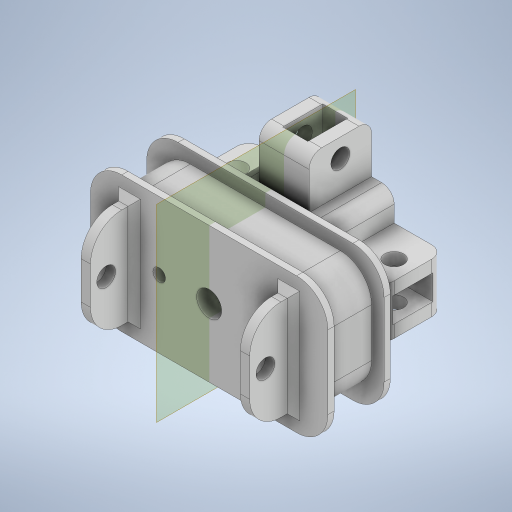
# Autodesk Inventor part: saw_end_v2
Saved by Autodesk Inventor 2024.3 (Build 283343000, 343)
## iProperties
Created: 2024-09-10
Part Number: saw_end_v2
Material: Generic
Document SubType Name: Modeling
Designer: magn1
Density: 1 g/cm^3
Appearance: Default
Author: magn1
Autodesk Inventor part; units mm, degrees
ref_plane "YZ Plane" through (0, 0, 0) normal (1, 0, 0) x (0, 1, 0)
ref_plane "XZ Plane" through (0, 0, 0) normal (0, 1, 0) x (-1, 0, 0)
ref_plane "XY Plane" through (0, 0, 0) normal (0, 0, 1) x (1, 0, 0)
sketch "Sketch1" plane through (0, 0, 0) normal (0, 0, 1) x (1, 0, 0)
  line L0 (-17, -8.875) -> (17, -8.875)
  line L1 (17, -8.875) -> (17, 8.875)
  line L2 (17, 8.875) -> (-17, 8.875)
  line L3 (-17, 8.875) -> (-17, -8.875)
  line L4 (-17, -8.875) -> (17, 8.875) construction
  line L5 (17, -8.875) -> (-17, 8.875) construction
  point P0 (0, 0)
  dimension "d0" = 34
  dimension "d1" = 17.75
  constraints: 12 end point, 2 midpoint, 2 parallel, 1 horizontal, 1 perpendicular
  measures "d0" distance of L2.end L1.end
  measures "d1" distance of L1.end L0.end
extrude "Extrusion1" add sketch "Sketch1" along normal blind 8
sketch "Sketch2" plane through (0, 0, 8) normal (0, 0, 1) x (1, 0, 0)
  line L0 (-19, -10.875) -> (19, -10.875)
  line L1 (19, -10.875) -> (19, 10.875)
  line L2 (19, 10.875) -> (-19, 10.875)
  line L3 (-19, 10.875) -> (-19, -10.875)
  line L4 (-19, -10.875) -> (19, 10.875) construction
  line L5 (19, -10.875) -> (-19, 10.875) construction
  point P0 (0, 0)
  dimension "d6" = 38
  dimension "d7" = 21.75
  constraints: 12 end point, 2 midpoint, 2 parallel, 1 horizontal, 1 perpendicular
  measures "d6" distance of L2.end L1.end
  measures "d7" distance of L1.end L0.end
extrude "Extrusion2" add sketch "Sketch2" along normal blind 1
sketch "Sketch3" plane through (0, 0, 0) normal (0, 0, -1) x (-1, 0, 0)
  line L0 (-19, 10.875) -> (19, 10.875) projected
  line L1 (-19, -10.875) -> (19, -10.875)
  line L2 (19, -10.875) -> (19, 10.875)
  line L3 (19, 10.875) -> (-19, 10.875)
  line L4 (-19, 10.875) -> (-19, -10.875)
  line L5 (-19, -10.875) -> (19, 10.875) construction
  line L6 (19, -10.875) -> (-19, 10.875) construction
  point P0 (0, 0)
  constraints: 12 end point, 2 midpoint, 2 parallel, 1 horizontal, 1 perpendicular
extrude "Extrusion3" add sketch "Sketch3" along normal blind 1
fillet "Fillet1" radius 5 12 edges at (19, 10.875, 8.5) (19, 10.875, -0.5) (19, -10.875, -0.5) (19, -10.875, 8.5) (17, -8.875, 4) (17, 8.875, 4) (-19, 10.875, 8.5) (-19, 10.875, -0.5) (-19, -10.875, -0.5) (-19, -10.875, 8.5) (-17, 8.875, 4) (-17, -8.875, 4)
sketch "Sketch6" plane through (0, 0, -1) normal (0, 0, -1) x (-1, 0, 0)
  line L0 (7.625, 8.625) -> (-7.625, 8.625)
  line L1 (-7.625, 8.625) -> (-7.625, -8.625)
  line L2 (-7.625, -8.625) -> (7.625, -8.625)
  line L3 (7.625, -8.625) -> (7.625, 8.625)
  line L4 (7.625, 8.625) -> (-7.625, -8.625) construction
  line L5 (-7.625, 8.625) -> (7.625, -8.625) construction
  circle A0 centre (0, 0) radius 2 projected
  circle A1 centre (0, 0) radius 1.5
  dimension "d19" = 15.25
  dimension "d20" = 17.25
  dimension "d21" = 3
  constraints: 12 end point, 2 midpoint, 2 parallel, 1 centre point, 1 coincident, 1 horizontal, 1 perpendicular
  measures "d19" distance of L2.end L1.end
  measures "d20" distance of L1.end L0.end
  measures "d21" diameter of A1
extrude "Extrusion6" add sketch "Sketch6" along normal blind 12 contours L3 L2 L1 L0 | A0 | A1
fillet "Fillet3" radius 2 4 edges at (-7.625, -8.625, -7) (7.625, -8.625, -7) (7.625, 8.625, -7) (-7.625, 8.625, -7)
sketch "Sketch9" plane through (0, 0, 9) normal (0, 0, 1) x (1, 0, 0)
  line L0 (0, 0) -> (12, 0) construction
  line L1 (0, 0) -> (-12, 0) construction
  line L2 (-12, 0) -> (-13.5, 0)
  line L3 (-13.5, 0) -> (-13.5, 8)
  line L4 (-13.5, 8) -> (-12, 8)
  line L5 (-12, 8) -> (-12, 0)
  line L6 (-13.5, 0) -> (-12, 0)
  line L7 (-12, 0) -> (-12, -8)
  line L8 (-12, -8) -> (-13.5, -8)
  line L9 (-13.5, -8) -> (-13.5, 0)
  line L10 (12, 0) -> (13.5, 0)
  line L11 (13.5, 0) -> (13.5, 8)
  line L12 (13.5, 8) -> (12, 8)
  line L13 (12, 8) -> (12, 0)
  line L14 (12, 0) -> (13.5, 0)
  line L15 (13.5, 0) -> (13.5, -8)
  line L16 (13.5, -8) -> (12, -8)
  line L17 (12, -8) -> (12, 0)
  dimension "d40" = 12
  dimension "d41" = 12
  dimension "d42" = 1.5
  dimension "d43" = 8
  dimension "d44" = 1.5
  dimension "d45" = 8
  dimension "d46" = 1.5
  dimension "d47" = 8
  dimension "d48" = 1.5
  dimension "d49" = 8
  constraints: 36 end point, 8 parallel, 6 horizontal, 4 perpendicular
  measures "d40" distance of L0.start L0.end
  measures "d41" distance of L0.start L1.end
  measures "d42" distance of L3.end L4.end
  measures "d43" distance of L2.end L3.end
  measures "d44" distance of L7.end L8.end
  measures "d45" distance of L6.end L7.end
  measures "d46" distance of L12.end L11.end
  measures "d47" distance of L11.end L10.end
  measures "d48" distance of L15.end L16.end
  measures "d49" distance of L14.end L15.end
extrude "Extrusion9" add sketch "Sketch9" along normal blind 7
sketch "Sketch11" plane through (13.5, -8, 9) normal (1, 0, 0) x (0, 0, -1)
  line L0 (-7, 16) -> (-7, 0) projected
  line L1 (-7, 8) -> (-4.5, 8) construction
  circle A0 centre (-4.5, 8) radius 1.5
  point P0 (9, 8)
  dimension "d52" = 2.5
  dimension "d53" = 3
  constraints: 2 end point, 1 centre point, 1 coincident, 1 horizontal, 1 midpoint
  measures "d52" distance of L1.start L1.end
  measures "d53" diameter of A0
extrude "Extrusion10" cut sketch "Sketch11" against normal up to surface (27 mm away)
fillet "Fillet4" radius 5 4 edges at (-12.75, 8, 16) (-12.75, -8, 16) (12.75, 8, 16) (12.75, -8, 16)
chamfer "Chamfer1" distance 1 angle 45 8 edges at (-13.5, 0, 9) (-12.75, -8, 9) (-12, 0, 9) (-12.75, 8, 9) (13.5, 0, 9) (12.75, 8, 9) (12, 0, 9) (12.75, -8, 9)
sketch "Sketch12" plane through (0, 0, 9) normal (0, 0, 1) x (1, 0, 0)
  circle A0 centre (0, 0) radius 2
  line L0 (0, 0) -> (8, 0) construction
  line L1 (0, 0) -> (-8, 0) construction
  circle A1 centre (-8, 0) radius 1
  circle A2 centre (8, 0) radius 1
  dimension "d73" = 4
  dimension "d74" = 8
  dimension "d75" = 8
  dimension "d76" = 2
  dimension "d77" = 2
  constraints: 4 end point, 3 centre point, 3 coincident, 2 horizontal
  measures "d73" diameter of A0
  measures "d74" distance of L0.start L0.end
  measures "d75" distance of L0.start L1.end
  measures "d76" diameter of A1
  measures "d77" diameter of A2
extrude "Extrusion11" cut sketch "Sketch12" against normal blind 6 contours A0
sketch "Sketch13" plane through (0, 0, -13) normal (0, 0, -1) x (-1, 0, 0)
  circle A0 centre (0, 0) radius 1.5
  dimension "d80" = 3
  constraints: 1 centre point, 1 coincident
  measures "d80" diameter of A0
extrude "Extrusion12" cut sketch "Sketch13" against normal blind 6
sketch "Sketch14" plane through (0, 0, -7) normal (0, 0, -1) x (-1, 0, 0)
  circle A0 centre (0, 0) radius 1.5
  dimension "d87" = 3
  constraints: 1 centre point, 1 coincident
  measures "d87" diameter of A0
loft "Loft2" cut profiles "Sketch14", "Sketch12" contours all / A2
loft "Loft3" cut profiles "Sketch14", "Sketch12" contours all / A1
sketch "Sketch15" plane through (-5.625, 8.625, -1) normal (0, 1, 0) x (1, 0, 0)
  line L0 (4.125, 12) -> (7.125, 12) construction
  line L1 (5.625, 12) -> (5.625, 2) construction
  line L2 (5.625, 6) -> (5.625, 3.1765) construction
  line L3 (5.625, 7) -> (2.625, 7) construction
  line L4 (5.625, 7) -> (8.625, 7) construction
  line L5 (5.625, 7) -> (8.625, 7) construction
  line L6 (1.625, 12) -> (3.625, 12)
  line L7 (3.625, 12) -> (3.625, 2)
  line L8 (3.625, 2) -> (1.625, 2)
  line L9 (1.625, 2) -> (1.625, 12)
  line L10 (1.625, 12) -> (3.625, 2) construction
  line L11 (3.625, 12) -> (1.625, 2) construction
  line L12 (9.625, 12) -> (7.625, 12)
  line L13 (7.625, 12) -> (7.625, 2)
  line L14 (7.625, 2) -> (9.625, 2)
  line L15 (9.625, 2) -> (9.625, 12)
  line L16 (9.625, 12) -> (7.625, 2) construction
  line L17 (7.625, 12) -> (9.625, 2) construction
  line L18 (1.625, 12) -> (9.625, 12)
  line L19 (9.625, 12) -> (9.625, 10.2)
  line L20 (9.625, 10.2) -> (1.625, 10.2)
  line L21 (1.625, 10.2) -> (1.625, 12)
  line L22 (1.625, 2) -> (9.625, 2)
  line L23 (9.625, 2) -> (9.625, 3.8)
  line L24 (9.625, 3.8) -> (1.625, 3.8)
  line L25 (1.625, 3.8) -> (1.625, 2)
  point P0 (5.625, -1)
  point P1 (3.625, 10.2)
  point P2 (7.625, 10.2)
  point P3 (7.625, 3.8)
  point P4 (3.625, 3.8)
  point P5 (3.625, 2)
  point P6 (7.625, 2)
  dimension "d121" = 8
  dimension "d96" = 10
  dimension "d97" = 3
  dimension "d98" = 180
  dimension "d99" = 3
  dimension "d100" = 2
  dimension "d101" = 10
  dimension "d102" = 2
  dimension "d103" = 10
  dimension "d111" = 8
  dimension "d112" = 1.8
  dimension "d113" = 8
  dimension "d114" = 1.8
  constraints: 48 end point, 8 parallel, 6 horizontal, 6 midpoint, 4 perpendicular, 3 collinear
  measures "d96" distance of L1.start L1.end
  measures "d97" distance of L3.start L3.end
  measures "d98" angle of L3 L4
  measures "d99" distance of L3.start L4.end
  measures "d100" distance of L7.end L8.end
  measures "d101" distance of L6.end L7.end
  measures "d102" distance of L14.end L13.end
  measures "d103" distance of L13.end L12.end
  measures "d111" distance of L19.end L20.end
  measures "d112" distance of L18.end L19.end
  measures "d113" distance of L24.end L23.end
  measures "d114" distance of L23.end L22.end
extrude "Extrusion13" add sketch "Sketch15" along normal blind 8 contours L6 L7 L20 L9 | L18 L13 L20 L7 | L20 L7 L24 L9 | L12 L15 L20 L13 | L24 L7 L8 L9 | L24 L13 L22 L7 | L20 L15 L24 L13 | L24 L15 L14 L13
sketch "Sketch16" plane through (4, 8.625, -3) normal (1, 0, 0) x (0, 0, -1)
  line L0 (10, 8) -> (0, 8) construction
  line L1 (5, 8) -> (5, 5) construction
  circle A0 centre (5, 5) radius 1.5
  point P0 (-3, -8.625)
  dimension "d106" = 3
  dimension "d107" = 3
  constraints: 2 end point, 1 centre point, 1 coincident, 1 midpoint, 1 vertical
  measures "d106" distance of L1.start L1.end
  measures "d107" diameter of A0
extrude "Extrusion14" cut sketch "Sketch16" against normal through all
fillet "Fillet5" radius 2 2 edges at (0, 16.625, -13) (0, 16.625, -3)
sketch "Sketch17" plane through (-7.625, -6.625, -1) normal (-1, 0, 0) x (0, 0, 1)
  line L0 (-12, 0) -> (-12, 13.25) projected
  line L1 (-12, 10.625) -> (-2, 10.625)
  line L2 (-2, 10.625) -> (-2, 8.625)
  line L3 (-2, 8.625) -> (-12, 8.625)
  line L4 (-12, 8.625) -> (-12, 10.625)
  line L5 (-12, 4.625) -> (-2, 4.625)
  line L6 (-2, 4.625) -> (-2, 2.625)
  line L7 (-2, 2.625) -> (-12, 2.625)
  line L8 (-12, 2.625) -> (-12, 4.625)
  line L9 (-12, 2.625) -> (-10.2, 2.625)
  line L10 (-10.2, 2.625) -> (-10.2, 10.625)
  line L11 (-10.2, 10.625) -> (-12, 10.625)
  line L12 (-12, 10.625) -> (-12, 2.625)
  line L13 (-2, 10.625) -> (-3.8, 10.625)
  line L14 (-3.8, 10.625) -> (-3.8, 2.625)
  line L15 (-3.8, 2.625) -> (-2, 2.625)
  line L16 (-2, 2.625) -> (-2, 10.625)
  point P0 (1, 6.625)
  point P1 (-12, 6.625)
  point P2 (-12, 2.625)
  point P3 (-2, 4.625)
  point P4 (-3.8, 8.625)
  point P5 (-3.8, 4.625)
  point P6 (-10.2, 4.625)
  point P7 (-10.2, 8.625)
  dimension "d115" = 10
  dimension "d116" = 2
  dimension "d117" = 10
  dimension "d118" = 2
  dimension "d119" = 4
  dimension "d120" = 2
  dimension "d128" = 1.8
  dimension "d129" = 8
  dimension "d130" = 1.8
  dimension "d131" = 8
  constraints: 32 end point, 8 parallel, 4 horizontal, 4 perpendicular, 2 point on line, 1 midpoint
  measures "d115" distance of L2.end L3.end
  measures "d116" distance of L1.end L2.end
  measures "d117" distance of L6.end L7.end
  measures "d118" distance of L5.end L6.end
  measures "d119" distance between parallel lines of L5 L3
  measures "d120" distance from line of L5 point (-12, 6.625)
  measures "d128" distance of L11.end L10.end
  measures "d129" distance of L10.end L9.end
  measures "d130" distance of L15.end L14.end
  measures "d131" distance of L14.end L13.end
extrude "Extrusion15" add sketch "Sketch17" along normal blind 8 contours L0 L5 L10 L7 | L0 L3 L10 L5 | L10 L5 L14 L7 | L0 L1 L10 L3 | L14 L5 L6 L7 | L10 L1 L14 L3 | L14 L3 L16 L5 | L14 L1 L2 L3
sketch "Sketch18" plane through (-7.625, 4, -3) normal (0, 1, 0) x (1, 0, 0)
  line L0 (-8, 0) -> (-8, 10) construction
  line L1 (-8, 5) -> (-5, 5) construction
  circle A0 centre (-5, 5) radius 1.5
  point P0 (7.625, -3)
  dimension "d123" = 3
  dimension "d124" = 3
  constraints: 2 end point, 1 centre point, 1 coincident, 1 horizontal, 1 midpoint
  measures "d123" distance of L1.start L1.end
  measures "d124" diameter of A0
extrude "Extrusion16" cut sketch "Sketch18" against normal through all
fillet "Fillet7" radius 2 2 edges at (-15.625, 0, -13) (-15.625, 0, -3)
ref_plane "Work Plane1" through (0, -6.625, -1) normal (-1, 0, 0) x (0, 0, 1)
mirror "Mirror1" about plane through (0, -6.625, -1) normal (-1, 0, 0) of "Extrusion15", "Extrusion16", "Fillet7"
body "Solid1"
